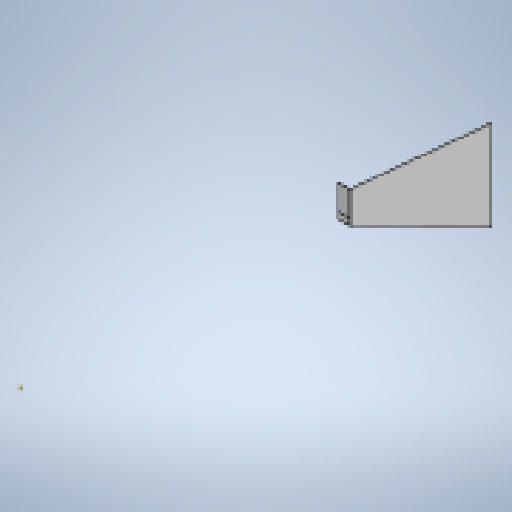
# Autodesk Inventor part: MSC 502 sheet belly-neck
Saved by Autodesk Inventor 2025 (Build 290162010, 162A)
## iProperties
Created: 2024-04-28
Part Number: MSC 502 sheet belly-neck
Material: Stainless Steel
Document SubType Name: Sheet Metal
Designer: admin
Mass: 38113.6 g
Surface Area: 31958.5 cm^2
Volume: 4764.2 cm^3
Density: 8 g/cm^3
Flat Pattern Width: 79.4949 cm
Flat Pattern Length: 134.83 cm
Flat Pattern Area: 10718.3 cm^2
Sheet Metal Rule: Default_mm
Sheet Metal Width: 794,949 mm
Sheet Metal Length: 1348,299 mm
Sheet Metal Area: 1071828,025 mm^2
Appearance: Default
Stock Number: МОО 502 лист брюхо-горло
Author: admin
Autodesk Inventor part; units mm, degrees
ref_plane "YZ Plane" through (0, 0, 0) normal (1, 0, 0) x (0, 1, 0)
ref_plane "XZ Plane" through (0, 0, 0) normal (0, 1, 0) x (-1, 0, 0)
ref_plane "XY Plane" through (0, 0, 0) normal (0, 0, 1) x (1, 0, 0)
sketch "Sketch1" plane through (0, 0, 0) normal (0, 0, 1) x (1, 0, 0)
  arc A0 (102, 0) -> (106.168, 1.684) centre (102, 6) ccw
  line L0 (106.168, 1.684) -> (744.2224, 617.8459)
  line L1 (-102, 0) -> (102, 0)
  point P0 (0, 0)
  point P1 (0, 0)
  dimension "d73" = 6
  dimension "d74" = 846.2224
  dimension "d75" = 136
  dimension "d82" = 887
  dimension "d83" = 204
  measures "d73" radius of A0
  measures "d74" horizontal distance of L1.start L0.end
  measures "d75" angle of L1 L0
  measures "d82" distance of L0.start L0.end
  measures "d83" distance of L1.start L1.end
contour flange "Contour Flange1" sketch "Sketch1" thickness 3 bend radius 3 width 800 along (0, 0, 1) mid plane no both sides no wall seen from (0, 0, 0) lies toward (0, 1, 0) curves L1 A0 L0
bend "Bend1"
corner "Corner1"
sketch "Sketch7" plane through (0, 0, 0) normal (1, 0, 0) x (0, 1, 0)
  line L0 (0, 800) -> (0, 0) projected
  line L1 (0, 0) -> (0, 800) projected
  line L2 (620.004, 0) -> (620.004, 800) projected
  line L3 (620.004, 800) -> (0, 800)
  line L4 (620.004, 800) -> (0, 279.7549)
  point P0 (0, 800)
  point P1 (0, 279.7549)
  dimension "d84" = 40
  constraints: 4 end point, 1 horizontal, 1 point on line
  measures "d84" angle of L3 L4
extrude "Extrusion3" cut sketch "Sketch7" along normal through all both and the other way through all
equation "\"d7\" = Thickness"
equation "\"d8\" = BendReliefWidth"
equation "\"d9\" = BendReliefDepth"
equation "\"d10\" = MinimumRemnant"
equation "\"d11\" = TransitionRadius"
equation "\"d13\" = BendRadius"
equation "\"d15\" = CornerReliefSize"
equation "\"d16\" = GapSize"
equation "\"d17\" = JacobiRadiusSize"
equation "\"BendRadius\" = Thickness"
equation "\"BendReliefWidth\" = Thickness"
equation "\"BendReliefDepth\" = 0.5 * Thickness"
equation "\"CornerReliefSize\" = 4 * Thickness"
equation "\"MinimumRemnant\" = 2 * Thickness"
equation "\"TransitionRadius\" = BendRadius"
equation "\"JacobiRadiusSize\" = BendRadius"
equation "\"GapSize\" = Thickness"
equation "\"d38\" = d40 + d44"
equation "\"d39\" = d40"
equation "\"d44\" = d40"
equation "\"Thickness\" = 3"
equation "\"d40\" = 3"
body "Solid1"
